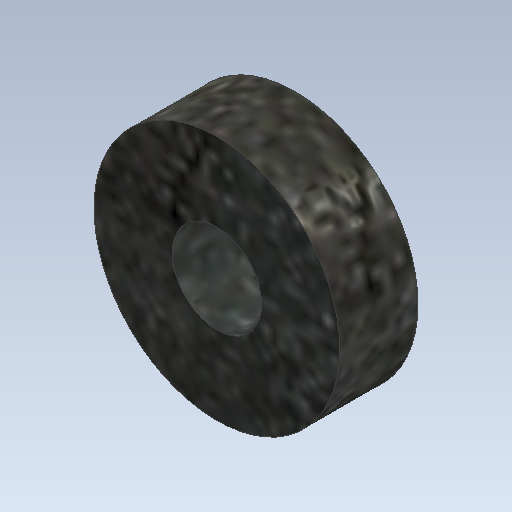
# Autodesk Inventor part: BEARINGSTANDIN
Saved by Autodesk Inventor 2020 (Build 240168000, 168)
## iProperties
Created: 2021-01-22
Part Number: BEARINGSTANDIN
Material: Steel
Document SubType Name: Modeling
Designer: lucky
Density: 7.85 g/cm^3
Appearance: Plate
Mass: 18.1262 g
Surface Area: 13.1947 cm^2
Volume: 2.30907 cm^3
Author: lucky
Autodesk Inventor part; units mm, degrees
ref_plane "YZ Plane" through (0, 0, 0) normal (1, 0, 0) x (0, 1, 0)
ref_plane "XZ Plane" through (0, 0, 0) normal (0, 1, 0) x (-1, 0, 0)
ref_plane "XY Plane" through (0, 0, 0) normal (0, 0, 1) x (1, 0, 0)
sketch "Sketch1" plane through (0, 0, 0) normal (0, 0, 1) x (1, 0, 0)
  circle A0 centre (0, 0) radius 4
  circle A1 centre (0, 0) radius 11
  dimension "d0" = 8
  dimension "d1" = 22
  constraints: 2 centre point, 2 coincident
  measures "d0" diameter of A0
  measures "d1" diameter of A1
extrude "Extrusion1" add sketch "Sketch1" along normal blind 7
body "Solid1"
